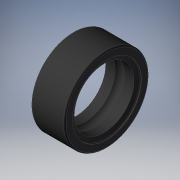
# Autodesk Inventor part: SKF_623-2RS1_or
Saved by Autodesk Inventor 2019 (Build 230136000, 136)
## iProperties
Created: 2023-07-31
Part Number: SKF_623-2RS1_or
Material: Generic
Catalog Web Link: www.cadenas.de
Description: BB1_001_101_or-Deep groove ball bearings
Vendor: SKF
Document SubType Name: Modeling
Designer: psAdmin
Manufacturer: SKF
Mass: 0.144489 g
Surface Area: 2.95757 cm^2
Volume: 0.144489 cm^3
Density: 1 g/cm^3
Appearance: PSOLRGB-175-175-175
Category: PARTsolutions
Company: SKF
Title: SKF_623-2RS1_or
Author: Cadenas PARTsolutions
Comments: Deep groove ball bearings
PSOL_IDENT_0: {$CADENAS_DATA/23d-libs/skf/bearings_units_and_housings/ball_bearings/deep_groove_ball_bearings/part
PSOL_IDENT_1: s/bb1_001_101_or.prj},181 {VTYP=3D},{NB=SKF_623-2RS1_or},{LINA=SKF_623-2RS1_or},{NN=BB1_001_101_or},
PSOL_IDENT_2: {DATE=25.11.2022 05:56:16},{GEOMDATE=21.11.2022 10:24:00},{VERSION=},{LINEID=11110},{WBVAR=},{WBNUME
PSOL_IDENT_3: RIC=}  {NB=SKF_623-2RS1_or},{LINA=SKF_623-2RS1_or},{KT=DUMMY},{DESIGNATION=623-2RS1},{R12=0.15},{DD=
PSOL_IDENT_4: 3.000},{D=10.000},{B=4.000},{C=},{CX=},{CXX=},{CA=0.000},{XXVARIANT=},{XXDESIGN=Single row},{XXSEALI
PSOL_IDENT_5: NG=Contact seal on both sides},{DESIGN=dgbbrs},{DESIGNIR=dgbbrs},{VARIANT=},{DD1=4.80},{DD2=},{DD2X=
PSOL_IDENT_6: },{DD2A=0.00},{D1=7.08},{D1X=0.00},{D2=8.2},{D2A=8.20},{D3=},{D3X=},{D3A=0.000},{D4=},{HH=0.000},{BB=
PSOL_IDENT_7: 0.000},{BBX=},{BBA=0.000},{FF=},{R0MAX=0.000},{R0=0.000},{PITCH=5.94},{DW=1.588},{DDAMIN=4.200},{DDA
PSOL_IDENT_8: MAX=5.100},{DDBMIN=0.000},{DDBMAX=0.000},{DBMIN=0.000},{DAMAX=8.800},{BBAMIN=0.000},{CAMAX=0.000},{R
PSOL_IDENT_9: AMAX=0.100},{LOAD1=0.540},{LOAD2=0.180},{LOAD3=0.007},{SPEED1=0},{SPEED2=40000},{KR=0.025},{F0=7.500
PSOL_IDENT_10: },{Z=7},{II=1},{MASS=0.002},{BEARING=623-2RS1},{RING=},{HELP=1.460},{HELP2=0.900},{DD1ALG=2.400},{YA
PSOL_IDENT_11: LG=2.400},{PITCH1=5.940},{DW1=1.588},{YALG1=3.540},{HALG1=1.460},{SH=2.400},{CU=0.482},{HALG=0.9},{B
PSOL_IDENT_12: 1=0},{SHIELDHELP=2},{D4A=0.000},{FFA=0.000},{RS1=X},{HELP3=0},{SUPPRESS=0}
NB: SKF_623-2RS1_or
NN: BB1_001_101_or
NT: Deep groove ball bearings
NBSYN: SKF_$DESIGNATION._or
LINA: SKF_623-2RS1_or
CATALOG: SKF
DESIGNATION: 623-2RS1
R12: 0.15
DD: 3
D: 10
B: 4
XXDESIGN: Single row
XXSEALING: Contact seal on both sides
DD1: 4.8
D1: 7.08
D1X: 0
D2: 8.2
HH: 0
BB: 0
R0MAX: 0
R0: 0
PITCH: 5.94
DW: 1.588
DDAMIN: 4.2
DDAMAX: 5.1
DDBMIN: 0
DDBMAX: 0
DBMIN: 0
DAMAX: 8.8
BBAMIN: 0
CAMAX: 0
RAMAX: 0.1
LOAD1: 0.54
LOAD2: 0.18
LOAD3: 0.007
SPEED1: 0
SPEED2: 40000
KR: 0.025
F0: 7.5
Z: 7
II: 1
MASS: 0.002
BEARING: 623-2RS1
HELP3: 0
SUPPRESS: 0
SUPPLIER: SKF
ARTICLENO: SKF_623-2RS1_or
BOMINFO: SKF_623-2RS1_or
CREATOR: CADENAS GmbH
Autodesk Inventor part; units mm, degrees
ref_plane "YZ Plane" through (0, 0, 0) normal (1, 0, 0) x (0, 1, 0)
ref_plane "XZ Plane" through (0, 0, 0) normal (0, 1, 0) x (-1, 0, 0)
ref_plane "XY Plane" through (0, 0, 0) normal (0, 0, 1) x (1, 0, 0)
sketch "Sketch_15" plane through (0, 0, 0) normal (0, 0, 1) x (1, 0, 0)
  line L0 (50, 0) -> (-50, 0)
  line L1 (0, 4.1) -> (0.045, 4.1)
  arc A0 (0.225, 4.1) -> (0.045, 4.1) centre (0.135, 4.1) ccw
  line L2 (0.225, 4.1) -> (0.3237, 3.54)
  line L3 (0.3237, 3.54) -> (1.4472, 3.54)
  arc A1 (2.5528, 3.54) -> (1.4472, 3.54) centre (2, 2.97) ccw
  line L4 (2.5528, 3.54) -> (3.6763, 3.54)
  line L5 (3.6763, 3.54) -> (3.775, 4.1)
  arc A2 (3.955, 4.1) -> (3.775, 4.1) centre (3.865, 4.1) ccw
  line L6 (3.955, 4.1) -> (4, 4.1)
  line L7 (4, 4.1) -> (4, 4.85)
  arc A3 (4, 4.85) -> (3.85, 5) centre (3.85, 4.85) ccw
  line L8 (3.85, 5) -> (0.15, 5)
  arc A4 (0.15, 5) -> (0, 4.85) centre (0.15, 4.85) ccw
  line L9 (0, 4.85) -> (0, 4.1)
  constraints: 20 end point, 10 point on circle, 5 centre point
revolve "Revolution1" add sketch "Sketch_15" angle 360 about axis through (50, 0, 0) along (1, 0, 0)
ref_plane "or_XY" through (0, 0, 0) normal (0, 0, 1) x (1, 0, 0)
ref_plane "or_YZ" through (0, 0, 0) normal (1, 0, 0) x (0, 1, 0)
ref_plane "or_ZX" through (0, 0, 0) normal (0, 1, 0) x (0, 0, 1)
body "Solid1"
